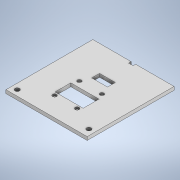
# Autodesk Inventor part: Box_cover
Saved by Autodesk Inventor 2021 (Build 250183000, 183)
## iProperties
Created: 2023-09-01
Part Number: Box_cover
Material: Genérico
Document SubType Name: Modeling
Designer: Sergio
Density: 1 g/cm^3
Appearance: Valor por defecto
Author: Sergio
Autodesk Inventor part; units mm, degrees
ref_plane "YZ Plane" through (0, 0, 0) normal (1, 0, 0) x (0, 1, 0)
ref_plane "XZ Plane" through (0, 0, 0) normal (0, 1, 0) x (-1, 0, 0)
ref_plane "XY Plane" through (0, 0, 0) normal (0, 0, 1) x (1, 0, 0)
sketch "Boceto1" plane through (0, 0, 0) normal (0, 1, 0) x (-1, 0, 0)
  line L0 (0, 0) -> (36, 0)
  line L1 (36, 0) -> (36, 0)
  line L2 (36, 0) -> (36, 77)
  line L3 (36, 77) -> (36, 77)
  line L4 (36, 77) -> (-36, 77)
  line L5 (-36, 77) -> (-36, 0)
  line L6 (-36, 0) -> (0, 0)
  line L7 (36, 77) -> (31, 77)
  line L8 (31, 77) -> (31, 72)
  line L9 (-36, 77) -> (-36, 75.5)
  line L10 (-36, 75.5) -> (-36, 70.5)
  line L11 (-36, 70.5) -> (-31, 70.5)
  circle A0 centre (-31, 70.5) radius 2
  circle A1 centre (31, 72) radius 2
  line L12 (36, 0) -> (0, 0)
  line L13 (0, 0) -> (0, 2.25)
  line L14 (0, 2.25) -> (2, 2.25)
  line L15 (2, 2.25) -> (2, 0)
  line L16 (0, 2.25) -> (-2, 2.25)
  line L17 (-2, 2.25) -> (-2, 0)
  line L18 (0, 0) -> (0, 50)
  line L19 (-12.5, 57) -> (12.5, 57)
  line L20 (12.5, 57) -> (12.5, 43)
  line L21 (12.5, 43) -> (-12.5, 43)
  line L22 (-12.5, 43) -> (-12.5, 57)
  line L23 (-12.5, 57) -> (12.5, 43) construction
  line L24 (12.5, 57) -> (-12.5, 43) construction
  line L25 (-12.5, 57) -> (12.5, 57)
  line L26 (12.5, 57) -> (12.5, 62.4)
  line L27 (12.5, 62.4) -> (-12.5, 62.4)
  line L28 (-12.5, 62.4) -> (-12.5, 57)
  line L29 (12.5, 62.4) -> (10, 62.4)
  line L30 (10, 62.4) -> (10, 59.9)
  line L31 (-12.5, 62.4) -> (-10, 62.4)
  line L32 (-10, 62.4) -> (-10, 59.9)
  circle A2 centre (10, 59.9) radius 1.75
  circle A3 centre (-10, 59.9) radius 1.75
  line L33 (-12.5, 62.4) -> (-12.5, 35.4)
  line L34 (-12.5, 35.4) -> (12.5, 35.4)
  line L35 (12.5, 35.4) -> (12.5, 62.4)
  line L36 (12.5, 62.4) -> (-12.5, 62.4)
  line L37 (-12.5, 35.4) -> (-10, 35.4)
  line L38 (-10, 35.4) -> (-10, 37.9)
  line L39 (12.5, 35.4) -> (12.5, 37.9)
  line L40 (12.5, 37.9) -> (10, 37.9)
  circle A4 centre (10, 37.9) radius 1.75
  circle A5 centre (-10, 37.9) radius 1.75
  circle A6 centre (31, 72) radius 4
  circle A7 centre (-31, 70.5) radius 4
  line L41 (0, 0) -> (0, 30)
  line L42 (0, 30) -> (0, 23)
  line L43 (0, 23) -> (7, 23)
  line L44 (7, 23) -> (7, 30)
  line L45 (7, 30) -> (-7, 30)
  line L46 (-7, 30) -> (-7, 23)
  line L47 (-7, 23) -> (0, 23)
  point P0 (2, 0)
  dimension "d0" = 36
  dimension "d1" = 0
  dimension "d2" = 77
  dimension "d3" = 0
  dimension "d4" = 72
  dimension "d5" = 5
  dimension "d6" = 5
  dimension "d7" = 1.5
  dimension "d8" = 5
  dimension "d9" = 5
  dimension "d10" = 4
  dimension "d11" = 4
  dimension "d14" = 36
  dimension "d15" = 2.25
  dimension "d16" = 2
  dimension "d17" = 2
  dimension "d18" = 50
  dimension "d19" = 25
  dimension "d20" = 14
  dimension "d21" = 5.4
  dimension "d22" = 2.5
  dimension "d23" = 2.5
  dimension "d24" = 2.5
  dimension "d25" = 2.5
  dimension "d26" = 3.5
  dimension "d27" = 3.5
  dimension "d28" = 27
  dimension "d29" = 25
  dimension "d30" = 2.5
  dimension "d31" = 2.5
  dimension "d32" = 2.5
  dimension "d33" = 2.5
  dimension "d34" = 3.5
  dimension "d35" = 3.5
  dimension "d50" = 8
  dimension "d51" = 8
  dimension "d61" = 30
  dimension "d63" = 7
  dimension "d64" = 14
  dimension "d65" = 7
  dimension "d66" = 0
  constraints: 96 end point, 20 perpendicular, 14 point on line, 8 centre point, 8 coincident, 6 parallel, 5 vertical, 3 horizontal, 2 midpoint
  measures "d0" distance of L0.start L0.end
  measures "d1" distance of L0.end L1.end
  measures "d2" distance of L1.end L2.end
  measures "d3" distance of L2.end L3.end
  measures "d4" distance of L3.end L4.end
  measures "d5" distance of L2.end L7.end
  measures "d6" distance of L7.end L8.end
  measures "d7" distance of L4.end L9.end
  measures "d8" distance of L9.end L10.end
  measures "d9" distance of L10.end L11.end
  measures "d10" diameter of A0
  measures "d11" diameter of A1
  measures "d14" distance of L0.end L12.end
  measures "d15" distance of L12.end L13.end
  measures "d16" distance of L13.end L14.end
  measures "d17" distance of L13.end L16.end
  measures "d18" distance of L12.end L18.end
  measures "d19" distance of L20.end L21.end
  measures "d20" distance of L19.end L20.end
  measures "d21" distance of L26.end L19.end
  measures "d22" distance of L26.end L29.end
  measures "d23" distance of L29.end L30.end
  measures "d24" distance of L27.end L31.end
  measures "d25" distance of L31.end L32.end
  measures "d26" diameter of A2
  measures "d27" diameter of A3
  measures "d28" distance of L27.end L33.end
  measures "d29" distance of L34.end L33.end
  measures "d30" distance of L33.end L37.end
  measures "d31" distance of L37.end L38.end
  measures "d32" distance of L34.end L39.end
  measures "d33" distance of L39.end L40.end
  measures "d34" diameter of A4
  measures "d35" diameter of A5
  measures "d50" diameter of A6
  measures "d51" diameter of A7
  measures "d61" distance of L12.end L41.end
  measures "d63" distance of L42.end L43.end
  measures "d64" distance between parallel lines of L46 L44
  measures "d65" distance between parallel lines of L43 L45
  measures "d66" distance from line of L41.end L45
extrude "Extrusión1" add sketch "Boceto1" against normal blind 3 contours L15 L14 L16 L17 L6 L5 L4 L2 L0 | L34 L33 L21 L18 | L18 L21 L35 L34 | L19 L28 L27 L26 | A2 | A3 | A4 | A5 | A6 | A7
extrude "Extrusión2" cut sketch "Boceto1" against normal blind 1.5 contours A2 | A3 | A4 | A5
thread "Rosca1" size "M4x0.7" class "6H" standard "ANSI Metric M Profile" full length
thread "Rosca2" size "M4x0.7" class "6H" standard "ANSI Metric M Profile" full length
thread "Rosca3" size "M3.5x0.6" class "6H" standard "ANSI Metric M Profile" full length
thread "Rosca4" size "M3.5x0.6" class "6H" standard "ANSI Metric M Profile" full length
thread "Rosca5" size "M3.5x0.6" class "6H" standard "ANSI Metric M Profile" full length
thread "Rosca6" size "M3.5x0.6" class "6H" standard "ANSI Metric M Profile" full length
extrude "Extrusión3" [suppressed]
equation "\"d0\" = 0.5 * box_in_width"
equation "\"d2\" = box_in_deep"
equation "\"d4\" = box_in_width"
equation "\"d5\" = offset + 0.5 * screw_Dhead"
equation "\"d6\" = offset + 0.5 * screw_Dhead"
equation "\"d7\" = thikness_box"
equation "\"d8\" = offset + 0.5 * screw_Dhead"
equation "\"d9\" = offset + 0.5 * screw_Dhead"
equation "\"d10\" = screw_d"
equation "\"d11\" = screw_d"
equation "\"d14\" = 0.5 * box_in_width"
equation "\"d15\" = 1.5 * thikness_box"
equation "\"d19\" = screen_width"
equation "\"d20\" = screen_height"
equation "\"d21\" = top_from_screen"
equation "\"d22\" = offset_screw_screen + 0.5 * screw_d_screen"
equation "\"d23\" = offset_screw_screen + 0.5 * screw_d_screen"
equation "\"d24\" = offset_screw_screen + 0.5 * screw_d_screen"
equation "\"d25\" = offset_screw_screen + 0.5 * screw_d_screen"
equation "\"d28\" = height_screen_total"
equation "\"d29\" = screen_width"
equation "\"d30\" = offset_screw_screen + 0.5 * screw_d_screen"
equation "\"d31\" = offset_screw_screen + 0.5 * screw_d_screen"
equation "\"d32\" = offset_screw_screen + 0.5 * screw_d_screen"
equation "\"d33\" = offset_screw_screen + 0.5 * screw_d_screen"
equation "\"d50\" = screw_Dhead"
equation "\"d51\" = screw_Dhead"
equation "\"d64\" = 2 * d63"
equation "\"d12\" = 2 * thikness_box"
equation "\"d36\" = deep_screw_screen"
equation "\"thikness\" = 2"
equation "\"offset\" = 1"
equation "\"r1\" = 5.55"
equation "\"r2o\" = 59.75"
equation "\"delta_y\" = 6"
equation "\"wire_d\" = 1"
equation "\"width_ang_spring\" = 5"
equation "\"spring_int_diam\" = 8.5"
equation "\"spring_ext_diam\" = 10.5"
equation "\"r3\" = 8.25"
equation "\"r3R\" = 4.75"
equation "\"r3T\" = 6.74537"
equation "\"alpha\" = 54.847297deg"
equation "\"alpha2\" = 270deg"
equation "\"theta3_recogido\" = 305.152703deg"
equation "\"delta_theta_3\" = 45deg"
equation "\"joint_width\" = 12"
equation "\"joint_radius\" = 7.75"
equation "\"shaft_width\" = 15"
equation "\"shaft_joint_diameter\" = 7.75"
equation "\"separation_space\" = 0.5"
equation "\"height_finger\" = 42"
equation "\"cell_screw_head_diameter\" = 4"
equation "\"cell_screw_diameter\" = 2"
equation "\"cell_space\" = 2"
equation "\"cell_width\" = 6"
equation "\"cell_theta_position\" = 60deg"
equation "\"cell_thikness\" = 1"
equation "\"cell_lenght\" = 37"
equation "\"cell_z_space\" = 5"
equation "\"wire_D\" = 2.3"
equation "\"width_link\" = 8"
equation "\"Dt\" = 1.05949"
equation "\"Djoint_shaft\" = 2.3"
equation "\"shaft_x\" = 1.45"
equation "\"shaft_y\" = 6.45"
equation "\"lenght_body_link\" = 186.05"
equation "\"lenght_bar_support\" = 201.65"
equation "\"wire_spring_d\" = 1"
equation "\"spring_int_d\" = 6"
equation "\"spring_lenght\" = 28"
equation "\"trigger_offset\" = 2"
equation "\"m2_theta2o\" = 107deg"
equation "\"m2_r2\" = 28"
equation "\"e\" = 9"
equation "\"So\" = 17"
equation "\"m2_theta3o\" = -30deg"
equation "\"m2_r3\" = 19.75"
equation "\"m2_delta_theta1\" = 15deg"
equation "\"m2_theta3f\" = -60deg"
equation "\"trigger_thumb_lenght\" = 6"
equation "\"width_r12\" = 8"
equation "\"m2_r1\" = 25.2"
equation "\"r3_thikness\" = 3.5"
equation "\"t_thikness\" = 3"
equation "\"tg_width\" = 4"
equation "\"pivot_screw_d\" = 4"
equation "\"pivot_diameter\" = 7"
equation "\"sj_diam_shaft\" = 6"
equation "\"sj_groove\" = 2"
equation "\"sj_groove_deep\" = 7"
equation "\"sj_head_D\" = 7"
equation "\"sj_head_d\" = 4.7464"
equation "\"sj_head_height\" = 5"
equation "\"sf_lenght\" = 9.5"
equation "\"sf_base\" = 3"
equation "\"sf_head_height\" = 3"
equation "\"sf_head_width\" = 4.5"
equation "\"sf_head_offset\" = 0.25"
equation "\"sf_head_grip_width\" = 2"
equation "\"sf_head_angle\" = 45deg"
equation "\"sf_thikness\" = 5"
equation "\"screw_Dhead\" = 8"
equation "\"screw_d\" = 4"
equation "\"screw_lenght\" = 12"
equation "\"screwJ_base_D\" = 9"
equation "\"screwJ_top_D\" = 13"
equation "\"gj_D\" = 6"
equation "\"gj_d\" = 4"
equation "\"gj_out_section\" = 6"
equation "\"box_in_deep\" = 77"
equation "\"box_in_width\" = 72"
equation "\"box_in_height\" = 35"
equation "\"thikness_box\" = 1.5"
equation "\"box_slim_slider_lenght\" = 116"
equation "\"sf_flex_separation\" = 38.66667"
equation "\"flex_separation_theta\" = 60deg"
equation "\"box_fat_slider_lenght\" = 67"
equation "\"int_width_slider\" = 2"
equation "\"ext_width_slider\" = 3.5"
equation "\"fat_width_slider\" = 2"
equation "\"slim_width_slider\" = 1.5"
equation "\"sfbox_width\" = 1.5"
equation "\"sfbox_tip_width\" = 2.5"
equation "\"sfbox_theta1\" = 60deg"
equation "\"sfbox_theta2\" = 45deg"
equation "\"agarradera_theta\" = 60deg"
equation "\"agarradera_width\" = 4"
equation "\"agarradera_position\" = 82.13077"
equation "\"screen_width\" = 25"
equation "\"screen_height\" = 14"
equation "\"screw_d_screen\" = 3"
equation "\"offset_screw_screen\" = 1"
equation "\"height_screen_total\" = 27"
equation "\"top_from_screen\" = 5.4"
equation "\"deep_screw_screen\" = 1.5"
